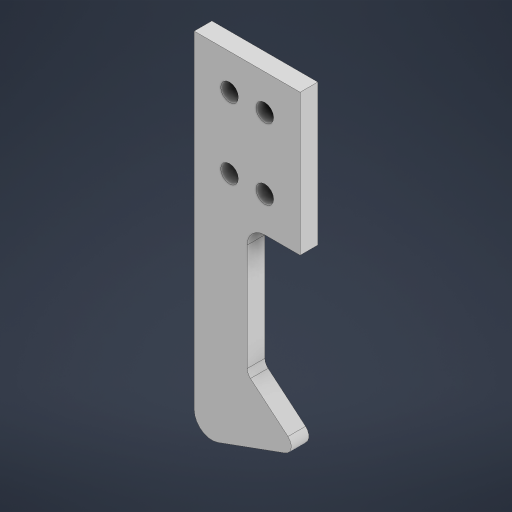
# Autodesk Inventor part: CS_Climb_Hooks
Saved by Autodesk Inventor 2023 (Build 270158000, 158)
## iProperties
Created: 2024-02-19
Part Number: CS_Climb_Hooks
Material: Generic
Document SubType Name: Modeling
Designer: kelle
Density: 1 g/cm^3
Appearance: Default
Author: kelle
Autodesk Inventor part; units mm, degrees
ref_plane "YZ Plane" through (0, 0, 0) normal (1, 0, 0) x (0, 1, 0)
ref_plane "XZ Plane" through (0, 0, 0) normal (0, 1, 0) x (-1, 0, 0)
ref_plane "XY Plane" through (0, 0, 0) normal (0, 0, 1) x (1, 0, 0)
sketch "Sketch1" plane through (0, 0, 0) normal (0, 0, 1) x (1, 0, 0)
  line L0 (9.525, -12.7) -> (-9.525, -12.7)
  line L1 (-9.525, -12.7) -> (-9.525, 12.7)
  line L2 (-9.525, 12.7) -> (9.525, 12.7)
  line L3 (9.525, 12.7) -> (9.525, -12.7)
  line L4 (9.525, -12.7) -> (-9.525, 12.7) construction
  line L5 (-9.525, -12.7) -> (9.525, 12.7) construction
  line L6 (-9.525, 12.7) -> (0, 12.7)
  line L7 (0, 12.7) -> (0, -50.8)
  line L8 (0, -50.8) -> (-9.525, -50.8)
  line L9 (-9.525, -50.8) -> (-9.525, 12.7)
  line L10 (-9.525, -50.8) -> (9.525, -43.8664)
  line L11 (-9.525, -50.8) -> (10.7476, -50.8) construction
  line L12 (9.525, -43.8664) -> (0, -35.8739)
  point P0 (0, 0)
  point P1 (0, -12.7)
  dimension "d0" = 19.05
  dimension "d1" = 25.4
  dimension "d2" = 63.5
  dimension "d3" = 20
  dimension "d4" = 60
  constraints: 26 end point, 4 parallel, 3 horizontal, 2 midpoint, 2 perpendicular, 1 equal length, 1 point on line
  measures "d0" distance of L1.end L2.end
  measures "d1" distance of L0.end L1.end
  measures "d2" distance of L6.end L7.end
  measures "d3" angle of L11 L10
  measures "d4" angle of L12 L10
extrude "Extrusion1" add sketch "Sketch1" along normal blind 3.175 contours L0 L7 L2 L3 | L7 L10 L9 L0 | L0 L1 L2 L7 | L12 L10 L7
sketch "Sketch2" plane through (0, 0, 3.175) normal (0, 0, 1) x (1, 0, 0)
  line L0 (-9.525, 12.7) -> (-9.525, -50.8) construction
  line L1 (-9.525, 0) -> (9.525, 0) construction
  line L2 (9.525, -12.7) -> (9.525, 12.7) construction
  line L3 (9.525, 12.7) -> (-9.525, 12.7) construction
  line L4 (0, -35.8739) -> (0, -12.7) construction
  line L5 (0, 12.7) -> (0, -12.7) construction
  circle A0 centre (3.175, 6.35) radius 1.5875
  circle A1 centre (3.175, -6.35) radius 1.5875
  circle A2 centre (-3.175, -6.35) radius 1.5875
  circle A3 centre (-3.175, 6.35) radius 1.5875
  line L6 (0, -12.7) -> (9.525, -12.7) projected
  point P0 (0, 0)
  dimension "d7" = 3.175
  dimension "d8" = 3.175
  dimension "d9" = 3.175
  dimension "d10" = 3.175
  dimension "d11" = 6.35
  dimension "d12" = 6.35
  dimension "d13" = 6.35
  dimension "d14" = 6.35
  dimension "d15" = 6.35
  dimension "d16" = 6.35
  dimension "d17" = 6.35
  dimension "d18" = 6.35
  dimension "d19" = 12.7
  constraints: 4 centre point, 4 end point, 2 midpoint, 1 point on line, 1 vertical
  measures "d7" diameter of A0
  measures "d8" diameter of A1
  measures "d9" diameter of A2
  measures "d10" diameter of A3
  measures "d11" distance from line of L3 A3.centre
  measures "d12" distance from line of L0 A3.centre
  measures "d13" distance from line of L3 A0.centre
  measures "d14" distance from line of L2 A0.centre
  measures "d15" distance from line of L2 A1.centre
  measures "d16" distance from line of L6 A1.centre
  measures "d17" distance from line of L0 A2.centre
  measures "d18" distance from line of L1 A2.centre
  measures "d19" distance between parallel lines of L3 L1
extrude "Extrusion2" cut sketch "Sketch2" against normal through all
fillet "Fillet1" radius 3.175 2 edges at (-9.525, -50.8, 1.5875) (0, -12.7, 1.5875)
fillet "Fillet2" radius 1.651 2 edges at (9.525, -43.8664, 1.5875) (0, -35.8739, 1.5875)
body "Solid1"
